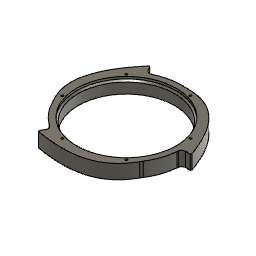
_Bottom ring.e895a1d6-2424-4fcb-819c-30bb705462ab (Autodesk Fusion 360 design; units mm, degrees)
Autodesk Fusion 360 part; units mm, degrees
sketch "Sketch1" plane through (0, 0, 0) normal (0, 1, 0) x (1, 0, 0)
  line L0 (-26.708, 42.6236) -> (-26.8379, 42.6236)
  line L1 (26.708, 42.6236) -> (27.1586, 42.6236)
  circle A0 centre (0, 0) radius 65
  circle A1 centre (0, 0) radius 67.15
  circle A2 centre (68.0978, 18.2467) radius 1.425
  line L2 (0, 0) -> (82, 0) construction
  line L3 (0, 0) -> (-41, 71.0141) construction
  line L4 (0, 0) -> (-41, -71.0141) construction
  line L5 (87.4769, -0.0257) -> (79.614, 0.0081)
  line L6 (-39.814, 68.9437) -> (-43.7162, 75.77)
  line L7 (-39.8, -68.9518) -> (-43.7607, -75.7444)
  line L8 (0, 0) -> (70.5, 0) construction
  arc A3 (79.614, 0.0081) -> (74.6944, -3.9877) centre (79.5926, -4.9919) ccw
  arc A4 (-39.814, 68.9437) -> (-33.8938, 66.6811) centre (-35.4732, 71.4251) ccw
  arc A5 (-39.8, -68.9518) -> (-40.8007, -62.6934) centre (-44.1194, -66.4332) ccw
  spline S0 degree 5 poles (-33.8938, 66.6811) (-33.483, 66.8179) (-33.0729, 66.9532) (-32.6634, 67.087) (-32.2547, 67.2193) (-31.8466, 67.3502) knots 0.021144 0.021144 0.021144 0.021144 0.021144 0.021144 0.032444 0.032444 0.032444 0.032444 0.032444 0.032444
  line L9 (-32.0549, 67.2834) -> (-31.6382, 67.417)
  spline S1 degree 5 poles (5.0849, 74.3263) (6.6179, 74.3731) (11.2429, 74.4207) (18.7539, 74.0099) (28.746, 72.2391) (40.5731, 67.6689) (52.3904, 59.5578) (62.916, 48.5693) (72.252, 34.9305) (78.8493, 22.0782) (83.3385, 11.4171) (86.1309, 3.8631) (87.4769, -0.0257) knots 0.251095 0.251095 0.251095 0.251095 0.251095 0.251095 0.3 0.4 0.5 0.6 0.7 0.8 0.9 1 1 1 1 1 1
  line L10 (-9.3123, 73.8863) -> (19.482, 74.7663)
  spline S2 degree 5 poles (-40.8007, -62.6934) (-41.1245, -62.4061) (-41.4467, -62.1186) (-41.7673, -61.8309) (-42.0863, -61.543) (-42.4037, -61.255) knots 0.021144 0.021144 0.021144 0.021144 0.021144 0.021144 0.032444 0.032444 0.032444 0.032444 0.032444 0.032444
  line L11 (-42.2416, -61.4021) -> (-42.5658, -61.1079)
  spline S3 degree 5 poles (-66.9109, -32.7595) (-67.718, -31.4553) (-70.0717, -27.4737) (-73.4714, -20.7636) (-76.9339, -11.2248) (-78.8895, 1.3029) (-77.7737, 15.5925) (-73.5202, 30.2022) (-66.3767, 45.1068) (-58.5449, 57.2464) (-51.5568, 66.4647) (-46.4109, 72.66) (-43.7162, 75.77) knots 0.251095 0.251095 0.251095 0.251095 0.251095 0.251095 0.3 0.4 0.5 0.6 0.7 0.8 0.9 1 1 1 1 1 1
  line L12 (-59.9171, -44.0611) -> (-73.9047, -21.4578)
  arc A6 (-66.9109, -32.7595) -> (-37.25, -64.5189) centre (0, 0) ccw
  spline S4 degree 5 poles (74.6944, -3.9877) (74.6075, -4.4118) (74.5196, -4.8346) (74.4308, -5.2561) (74.341, -5.6763) (74.2503, -6.0951) knots 0.021144 0.021144 0.021144 0.021144 0.021144 0.021144 0.032444 0.032444 0.032444 0.032444 0.032444 0.032444
  line L13 (74.2965, -5.8814) -> (74.204, -6.3089)
  spline S5 degree 5 poles (61.826, -41.5668) (61.1001, -42.9178) (58.8287, -46.947) (54.7175, -53.2463) (48.1879, -61.0143) (38.3164, -68.9717) (25.3834, -75.1503) (10.6042, -78.7715) (-5.8753, -80.0373) (-20.3044, -79.3246) (-31.7817, -77.8819) (-39.7199, -76.523) (-43.7607, -75.7444) knots 0.251095 0.251095 0.251095 0.251095 0.251095 0.251095 0.3 0.4 0.5 0.6 0.7 0.8 0.9 1 1 1 1 1 1
  line L14 (68.2252, -29.657) -> (55.4268, -53.4766)
  arc A7 (61.826, -41.5668) -> (74.5, 0) centre (0, 0) ccw
  arc A8 (5.0849, 74.3263) -> (-37.25, 64.5189) centre (0, 0) ccw
  circle A9 centre (18.2467, 68.0978) radius 1.425
  circle A10 centre (-49.851, 49.851) radius 1.425
  circle A11 centre (-68.0978, -18.2467) radius 1.425
  circle A12 centre (-18.2467, -68.0978) radius 1.425
  circle A13 centre (49.851, -49.851) radius 1.425
  line L15 (-15.6791, -68.6528) -> (-16.4822, -66.1517)
  line L16 (-16.4822, -66.1517) -> (-19.0499, -65.5966)
  line L17 (-19.0499, -65.5966) -> (-20.8144, -67.5427)
  line L18 (-20.8144, -67.5427) -> (-20.0113, -70.0439)
  line L19 (-20.0113, -70.0439) -> (-17.4436, -70.5989)
  line L20 (-17.4436, -70.5989) -> (-15.6791, -68.6528)
  line L21 (52.4187, -50.4061) -> (51.6155, -47.9049)
  line L22 (50.6541, -52.3522) -> (52.4187, -50.4061)
  line L23 (48.0865, -51.7971) -> (50.6541, -52.3522)
  line L24 (47.2834, -49.296) -> (48.0865, -51.7971)
  line L25 (49.0479, -47.3499) -> (47.2834, -49.296)
  line L26 (51.6155, -47.9049) -> (49.0479, -47.3499)
  line L27 (69.8623, 20.1928) -> (67.2947, 20.7479)
  line L28 (70.6654, 17.6917) -> (69.8623, 20.1928)
  line L29 (68.9009, 15.7456) -> (70.6654, 17.6917)
  line L30 (66.3333, 16.3006) -> (68.9009, 15.7456)
  line L31 (65.5301, 18.8018) -> (66.3333, 16.3006)
  line L32 (67.2947, 20.7479) -> (65.5301, 18.8018)
  line L33 (17.4436, 70.5989) -> (15.6791, 68.6528)
  line L34 (20.0113, 70.0439) -> (17.4436, 70.5989)
  line L35 (20.8144, 67.5427) -> (20.0113, 70.0439)
  line L36 (19.0499, 65.5966) -> (20.8144, 67.5427)
  line L37 (16.4822, 66.1517) -> (19.0499, 65.5966)
  line L38 (15.6791, 68.6528) -> (16.4822, 66.1517)
  line L39 (-52.4187, 50.4061) -> (-51.6155, 47.9049)
  line L40 (-50.6541, 52.3522) -> (-52.4187, 50.4061)
  line L41 (-48.0865, 51.7971) -> (-50.6541, 52.3522)
  line L42 (-47.2834, 49.296) -> (-48.0865, 51.7971)
  line L43 (-49.0479, 47.3499) -> (-47.2834, 49.296)
  line L44 (-51.6155, 47.9049) -> (-49.0479, 47.3499)
  line L45 (-69.8623, -20.1928) -> (-67.2947, -20.7479)
  line L46 (-70.6654, -17.6917) -> (-69.8623, -20.1928)
  line L47 (-68.9009, -15.7456) -> (-70.6654, -17.6917)
  line L48 (-66.3333, -16.3006) -> (-68.9009, -15.7456)
  line L49 (-65.5301, -18.8018) -> (-66.3333, -16.3006)
  line L50 (-67.2947, -20.7479) -> (-65.5301, -18.8018)
  point P0 (39, 67.55)
  point P1 (-78, 0)
  point P2 (39, -67.55)
  point P3 (-18.2467, -68.0978)
  dimension "d63" = 130
  dimension "d76" = 134.3
  dimension "d123" = 78
  dimension "d127" = 5
  dimension "d128" = 5
  dimension "d129" = 5
  dimension "d132" = 149
  dimension "d162" = 2.275
  dimension "d164" = 360
  constraint coincident A0.centre A1.centre
  constraint horizontal L2
  constraint horizontal L8
  constraint tangent A3 S4
  constraint tangent L5 A3
  constraint tangent A4 S0
  constraint tangent L6 A4
  constraint tangent A5 S2
  constraint tangent L7 A5
  constraint coincident S0.end A6
  constraint midpoint S0.end L9
  constraint coincident S1.start A6
  constraint midpoint S1.start L10
  constraint coincident L3 A8.end
  constraint coincident S2.end A6
  constraint midpoint S2.end L11
  constraint midpoint S3.start L12
  constraint coincident L4 A6.end
  constraint concentric A6 A7
  constraint coincident S4.end A7
  constraint midpoint S4.end L13
  constraint midpoint S5.start L14
  constraint coincident L2 A7.end
  constraint concentric A7 A8
  constraint coincident P3 A12.centre
  measures "d63" diameter of A0
  measures "d76" diameter of A1
  measures "d123" distance of A0.centre P0
  measures "d127" radius of A3
  measures "d128" radius of A4
  measures "d129" radius of A5
  measures "d132" diameter of A6
  measures "d162" distance of P3 L20
extrude "Extrude22" add sketch "Sketch1" against normal blind 19.1 contours A2 | L5 L6 L7 A3 A4 A5 S0 L9 S1 S2 L11 S3 A6 S4 L13 S5 A7 A8 | A9 | A10 | A11 | A12 | A13 | L15 L16 L17 L18 L19 L20 | L21 L22 L23 L24 L25 L26 | L27 L28 L29 L30 L31 L32 | L33 L34 L35 L36 L37 L38 | L39 L40 L41 L42 L43 L44 | L45 L46 L47 L48 L49 L50
extrude "Extrude23" add sketch "Sketch1" against normal blind 15.1 from surface at -4 contours A2 | A9 | A11 | A12 | A13 | L15 L16 L17 L18 L19 L20 | L21 L22 L23 L24 L25 L26 | L27 L28 L29 L30 L31 L32 | L33 L34 L35 L36 L37 L38 | L39 L40 L41 L42 L43 L44 | L45 L46 L47 L48 L49 L50
extrude "Extrude24" add sketch "Sketch1" against normal blind 19.1 contours A1
extrude "Extrude25" cut sketch "Sketch1" against normal blind 5.1 contours A1
chamfer "Chamfer3" distance 2.15 angle 45 1 edges at (-62.6058, -5.1, -24.2825)
fillet "Fillet2" radius 1 3 edges at (87.4769, -9.55, 0.0257) (-43.7607, -9.55, 75.7444) (-43.7162, -9.55, -75.77)
extrude "Extrude26" cut sketch "Sketch1" against normal blind 25 contours A2 | A9 | A10 | A11 | A12 | A13
fillet "Fillet3" radius 60 1 edges at (61.826, -9.55, 41.5668)
fillet "Fillet4" radius 60 1 edges at (-66.9109, -9.55, 32.7595)
fillet "Fillet5" radius 60 1 edges at (5.0849, -9.55, -74.3263)
extrude "Extrude27" cut sketch "Sketch1" against normal blind 20 contours L15 L16 L17 L18 L19 L20 | L21 L22 L23 L24 L25 L26 | L27 L28 L29 L30 L31 L32 | L33 L34 L35 L36 L37 L38 | L39 L40 L41 L42 L43 L44 | L45 L46 L47 L48 L49 L50
extrude "Extrude28" add sketch "Sketch1" against normal blind 16.6 contours L15 L16 L17 L18 L19 L20 | L21 L22 L23 L24 L25 L26 | L27 L28 L29 L30 L31 L32 | L33 L34 L35 L36 L37 L38 | L39 L40 L41 L42 L43 L44 | L45 L46 L47 L48 L49 L50
named bodies: "bottom ring"
